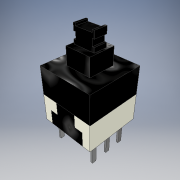
# Autodesk Inventor part: PushButton
Saved by Autodesk Inventor 2018 (Build 220112000, 112)
## iProperties
Created: 2021-02-07
Part Number: PushButton
Material: Všeobecné
Document SubType Name: Modeling
Designer: Jozko Mrkvicka
Density: 1 g/cm^3
Appearance: Výchozí
Author: Jozko Mrkvicka
Autodesk Inventor part; units mm, degrees
ref_plane "YZ Plane" through (0, 0, 0) normal (1, 0, 0) x (0, 1, 0)
ref_plane "XZ Plane" through (0, 0, 0) normal (0, 1, 0) x (-1, 0, 0)
sketch "Náčrt1" plane through (0, 0, 0) normal (0, 1, 0) x (-1, 0, 0)
  line L0 (0, 0) -> (8.255, 0)
  line L1 (8.255, 0) -> (8.255, -8.255)
  line L2 (8.255, -8.255) -> (0, -8.255)
  line L3 (0, -8.255) -> (0, 0)
  dimension "d0" = 8.255
  dimension "d1" = 8.255
  constraints: 8 end point, 2 parallel, 1 horizontal, 1 perpendicular
  measures "d0" distance of L1.end L2.end
  measures "d1" distance of L0.end L1.end
extrude "Vysunutí1" add sketch "Náčrt1" along normal blind 8.255
sketch "Náčrt2" plane through (0, 0, 0) normal (0, -1, 0) x (1, 0, 0)
  line L0 (0, 0) -> (-8.255, 0) projected
  line L1 (0, -8.255) -> (0, 0) projected
  line L2 (-0.7937, -1.27) -> (-1.1113, -1.27)
  line L3 (-1.1113, -1.27) -> (-1.1112, -1.905)
  line L4 (-1.1112, -1.905) -> (-0.7937, -1.905)
  line L5 (-0.7937, -1.905) -> (-0.7937, -1.27)
  line L6 (-0.7937, -3.81) -> (-1.1113, -3.81)
  line L7 (-1.1113, -3.81) -> (-1.1112, -4.445)
  line L8 (-1.1112, -4.445) -> (-0.7937, -4.445)
  line L9 (-0.7937, -4.445) -> (-0.7937, -3.81)
  line L10 (-0.7938, -6.35) -> (-1.1113, -6.35)
  line L11 (-1.1113, -6.35) -> (-1.1112, -6.985)
  line L12 (-1.1112, -6.985) -> (-0.7937, -6.985)
  line L13 (-0.7937, -6.985) -> (-0.7938, -6.35)
  line L14 (-7.1438, -1.27) -> (-7.4613, -1.27)
  line L15 (-7.4613, -1.27) -> (-7.4613, -1.905)
  line L16 (-7.4613, -1.905) -> (-7.1438, -1.905)
  line L17 (-7.1438, -1.905) -> (-7.1438, -1.27)
  line L18 (-7.1438, -3.81) -> (-7.4613, -3.81)
  line L19 (-7.4613, -3.81) -> (-7.4613, -4.445)
  line L20 (-7.4613, -4.445) -> (-7.1438, -4.445)
  line L21 (-7.1438, -4.445) -> (-7.1438, -3.81)
  line L22 (-7.1438, -6.35) -> (-7.4613, -6.35)
  line L23 (-7.4613, -6.35) -> (-7.4613, -6.985)
  line L24 (-7.4613, -6.985) -> (-7.1438, -6.985)
  line L25 (-7.1438, -6.985) -> (-7.1438, -6.35)
  point P0 (-4.1275, -4.1275)
  point P1 (-4.1275, -4.1275)
  dimension "d4" = 0.3175
  dimension "d5" = 0.635
  dimension "d8" = 2.54
  dimension "d11" = 6.35
  dimension "d15" = 8.255
  constraints: 48 end point, 2 horizontal, 2 parallel, 1 perpendicular, 1 vertical, 40 other
  measures "d4" distance of L4.end L3.end
  measures "d5" distance of L3.end L2.end
  measures "d8" distance of L2.start L6.start
  measures "d11" distance of L2.start L14.start
  measures "d15" distance of L0.start L0.end
extrude "Vysunutí2" add sketch "Náčrt2" along normal blind 3.81
sketch "Náčrt3" plane through (0, 8.255, 0) normal (0, 1, 0) x (1, 0, 0)
  line L0 (-6.0325, 2.2225) -> (-2.2225, 2.2225)
  line L1 (-2.2225, 2.2225) -> (-2.2225, 6.0325)
  line L2 (-2.2225, 6.0325) -> (-6.0325, 6.0325)
  line L3 (-6.0325, 6.0325) -> (-6.0325, 2.2225)
  line L4 (-6.0325, 2.2225) -> (-2.2225, 6.0325) construction
  line L5 (-2.2225, 2.2225) -> (-6.0325, 6.0325) construction
  point P0 (-4.1275, 4.1275)
  dimension "d18" = 3.81
  dimension "d19" = 3.81
  constraints: 12 end point, 2 midpoint, 2 parallel, 1 horizontal, 1 perpendicular
  measures "d18" distance of L2.end L1.end
  measures "d19" distance of L1.end L0.end
extrude "Vysunutí3" add sketch "Náčrt3" along normal blind 2.54
sketch "Náčrt4" plane through (0, 10.795, 0) normal (0, 1, 0) x (1, 0, 0)
  line L0 (-5.715, 3.175) -> (-2.54, 3.175)
  line L1 (-2.54, 3.175) -> (-2.54, 5.08)
  line L2 (-2.54, 5.08) -> (-5.715, 5.08)
  line L3 (-5.715, 5.08) -> (-5.715, 3.175)
  line L4 (-5.715, 3.175) -> (-2.54, 5.08) construction
  line L5 (-2.54, 3.175) -> (-5.715, 5.08) construction
  point P0 (0, 0)
  point P1 (-4.1275, 4.1275)
  dimension "d22" = 3.175
  dimension "d23" = 1.905
  constraints: 12 end point, 2 midpoint, 2 parallel, 1 horizontal, 1 perpendicular
  measures "d22" distance of L2.end L1.end
  measures "d23" distance of L1.end L0.end
extrude "Vysunutí4" add sketch "Náčrt4" along normal blind 2.54
sketch "Náčrt6" plane through (-5.715, 10.795, -3.175) normal (0, 0, 1) x (1, 0, 0)
  line L0 (0, 2.54) -> (3.175, 2.54) projected
  line L1 (0.3175, 2.2225) -> (2.8575, 2.2225)
  line L2 (2.8575, 2.2225) -> (2.8575, 2.54)
  line L3 (0.3175, 2.54) -> (0.3175, 2.2225)
  line L4 (0, 0.635) -> (0.3175, 0.635)
  line L5 (0.3175, 0.635) -> (0.3175, 1.5875)
  line L6 (3.175, 0.635) -> (2.8575, 0.635)
  line L7 (2.8575, 0.635) -> (2.8575, 1.5875)
  line L8 (0.3175, 2.54) -> (2.8575, 2.54)
  line L9 (3.175, 1.5875) -> (3.175, 0.635)
  line L10 (0, 1.5875) -> (0, 0.635)
  line L11 (0, 0) -> (0, 2.54) projected
  line L12 (0, 1.5875) -> (0.3175, 1.5875)
  line L13 (3.175, 0) -> (3.175, 2.54) projected
  line L14 (3.175, 1.5875) -> (2.8575, 1.5875)
  point P0 (5.715, -10.795)
  point P1 (1.5875, 2.54)
  constraints: 24 end point, 3 horizontal, 3 perpendicular, 3 point on line, 1 midpoint, 1 parallel
extrude "Vysunutí5" cut sketch "Náčrt6" against normal up to next
ref_plane "Pracovní rovina1" through (0, 4.1275, 0) normal (0, -1, 0) x (1, 0, 0)
split_face "Rozdělit1"
sketch "Náčrt7" plane through (-8.255, 0, 0) normal (0, 0, 1) x (1, 0, 0)
  line L0 (0, 4.1275) -> (8.255, 4.1275) projected
  line L1 (8.255, 0) -> (0, 0) projected
  line L2 (5.715, 4.1275) -> (5.715, 2.2225)
  line L3 (2.54, 2.2225) -> (2.54, 4.1275)
  line L4 (1.27, 0) -> (6.985, 0)
  line L5 (6.985, 0) -> (6.985, 2.2225)
  line L6 (1.27, 2.2225) -> (1.27, 0)
  line L7 (1.27, 2.2225) -> (2.54, 2.2225)
  line L8 (5.715, 2.2225) -> (6.985, 2.2225)
  line L9 (2.54, 4.1275) -> (5.715, 4.1275)
  point P0 (4.1275, 4.1275)
  point P1 (4.1275, 2.2225)
  constraints: 16 end point, 3 point on line, 2 parallel, 1 horizontal, 1 midpoint
split_face "Rozdělit2"
